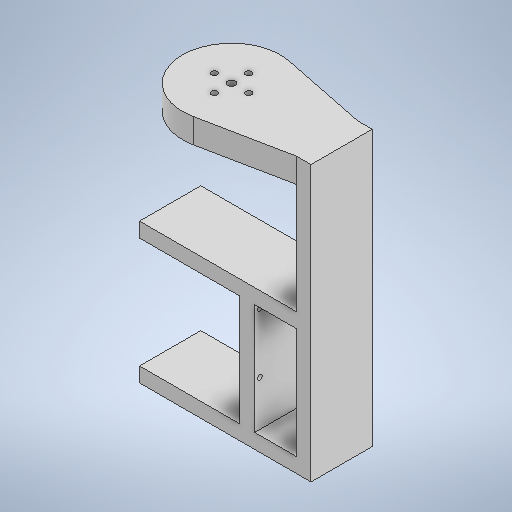
# Autodesk Inventor part: wahacz
Saved by Autodesk Inventor 2025.3 (Build 293356000, 356)
## iProperties
Created: 2026-03-17
Part Number: wahacz
Material: Generic
Document SubType Name: Modeling
Designer: ksawe
Density: 1 g/cm^3
Appearance: Default
Author: ksawe
Autodesk Inventor part; units mm, degrees
ref_plane "YZ Plane" through (0, 0, 0) normal (1, 0, 0) x (0, 1, 0)
ref_plane "XZ Plane" through (0, 0, 0) normal (0, 1, 0) x (-1, 0, 0)
ref_plane "XY Plane" through (0, 0, 0) normal (0, 0, 1) x (1, 0, 0)
sketch "Sketch1" plane through (0, 0, 0) normal (0, 0, 1) x (1, 0, 0)
  line L0 (0, -10.22) -> (0, 35)
  line L1 (0, -10.22) -> (-41, -10.22)
  line L2 (0, 35) -> (-41, 35)
  line L3 (-41, 41) -> (23, 41)
  line L4 (6, 35) -> (6, -10.22)
  line L5 (29, -16.22) -> (-41, -16.22)
  line L6 (-41, 41) -> (-41, 35)
  line L7 (-41, -10.22) -> (-41, -16.22)
  line L8 (-41, 41) -> (23, 41)
  line L9 (-41, -16.22) -> (29, -16.22)
  line L10 (29, -16.22) -> (29, 96)
  line L11 (23, 41) -> (-41, 41)
  line L12 (6, 35) -> (23, 35)
  line L13 (23, 35) -> (23, -10.22)
  line L14 (23, -10.22) -> (6, -10.22)
  line L15 (29, 41) -> (29, 96)
  line L16 (29, 96) -> (23, 96)
  line L17 (23, 96) -> (23, 41)
  line L18 (29, -16.22) -> (29, 96)
  point P0 (23, 41)
  dimension "d114" = 17
  dimension "d115" = 41
  dimension "d116" = 6
  dimension "d117" = 6
  dimension "d118" = 6
  dimension "d119" = 45.22
  dimension "d120" = 70
  dimension "d121" = 6
  dimension "d122" = 6
  dimension "d136" = 55
  constraints: 38 end point, 12 parallel, 1 collinear, 1 horizontal, 1 vertical
  measures "d114" distance of L4.start L12.end
  measures "d115" distance of L0.end L2.end
  measures "d116" distance between parallel lines of L4 L0
  measures "d117" distance of L3.start L2.end
  measures "d118" distance of L1.end L5.end
  measures "d119" distance of L0.start L0.end
  measures "d120" distance of L5.start L5.end
  measures "d121" distance of L10.end L16.end
  measures "d122" distance between parallel lines of L10 L13
  measures "d136" distance of L16.end L3.end
extrude "Extrusion1" add sketch "Sketch1" along normal blind 25
sketch "Sketch2" plane through (6, -16.22, 0) normal (1, 0, 0) x (0, 0, -1)
  line L0 (0, 57.22) -> (-25, 57.22) projected
  line L1 (0, 51.22) -> (-25, 51.22) projected
  line L2 (0, 6) -> (-25, 6) projected
  circle A0 centre (-22.89, 48.81) radius 1
  circle A1 centre (-22.89, 24.41) radius 1
  line L3 (0, 0) -> (-25, 0) projected
  line L4 (-25, 6) -> (-25, 51.22) projected
  line L5 (-12.5, 6) -> (-12.5, 51.22)
  circle A2 centre (-2.11, 48.81) radius 1
  circle A3 centre (-2.11, 24.41) radius 1
  point P0 (0, 16.22)
  point P1 (-25, 102.22)
  dimension "d19" = 2
  dimension "d20" = 2
  dimension "d21" = 24.4
  dimension "d24" = 18.41
  dimension "d25" = 2.11
  constraints: 4 centre point, 2 end point, 2 midpoint, 2 symmetric about line, 1 vertical alignment, 2 other
  measures "d19" diameter of A0
  measures "d20" diameter of A1
  measures "d21" distance of A1.centre A0.centre
  measures "d24" distance from line of L2 A1.centre
  measures "d25" distance from line of L4 A1.centre
extrude "Extrusion2" cut sketch "Sketch2" against normal blind 25 contours A0 | A1 | A2 | A3
sketch "Sketch3" plane through (23, 96, 0) normal (0, 1, 0) x (1, 0, 0)
  arc A0 (-35, 7.1443) -> (-35.0521, -32.058) centre (-39, -12.4516) ccw
  line L0 (0, 0) -> (0, -25) projected
  line L1 (6, 0) -> (0, 0) projected
  line L2 (0, 0) -> (-35, 7.1443)
  line L3 (0, -25) -> (-35.0521, -32.058)
  point P0 (-23, 0)
  dimension "d137" = 40
  dimension "d138" = 39
  dimension "d140" = 35
  constraints: 4 end point, 2 point on circle, 2 tangent, 1 centre point
  measures "d137" diameter of A0
  measures "d138" distance from line of L0 A0.centre
  measures "d140" horizontal distance of L2.end L0.start
extrude "Extrusion3" add sketch "Sketch3" against normal blind 10
sketch "Sketch13" plane through (29, 96, 25) normal (0, 1, 0) x (1, 0, 0)
  arc A0 (-41, 32.1443) -> (-41.0521, -7.058) centre (-45, 12.5484) ccw projected
  circle A1 centre (-45, 12.5484) radius 1.6
  circle A2 centre (-45, 19.5484) radius 1.25
  circle A3 centre (-52, 12.5484) radius 1.25
  circle A4 centre (-45, 5.5484) radius 1.25
  circle A5 centre (-38, 12.5484) radius 1.25
  point P0 (-29, 25)
  dimension "d218" = 3.2
  dimension "d219" = 2.5
  dimension "d222" = 360
  dimension "d224" = 7
  dimension "d225" = 7
  constraints: 5 centre point, 1 coincident, 9 other
  measures "d218" diameter of A1
  measures "d219" diameter of A2
  measures "d224" horizontal distance of A2.centre A5.centre
  measures "d225" distance of A5.centre A0.centre
extrude "Extrusion6" cut sketch "Sketch13" against normal blind 10
body "Solid1"
